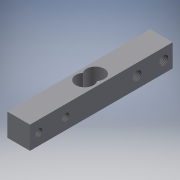
# Autodesk Inventor part: Celda
Saved by Autodesk Inventor 2019 (Build 230136000, 136)
## iProperties
Created: 2020-01-19
Part Number: Celda
Material: Generic
Document SubType Name: Modeling
Designer: peter
Density: 2.69895 g/cm^3
Appearance: Default
Mass: 28 g
Surface Area: 52.6894 cm^2
Volume: 10.3744 cm^3
Author: peter
Autodesk Inventor part; units mm, degrees
ref_plane "YZ Plane" through (0, 0, 0) normal (1, 0, 0) x (0, 1, 0)
ref_plane "XZ Plane" through (0, 0, 0) normal (0, 1, 0) x (-1, 0, 0)
ref_plane "XY Plane" through (0, 0, 0) normal (0, 0, 1) x (1, 0, 0)
sketch "Sketch1" plane through (0, 0, 0) normal (0, 1, 0) x (-1, 0, 0)
  line L0 (9.5195, 30.881) -> (-3.1805, 30.881)
  line L1 (-3.1805, 30.881) -> (-3.1805, -49.119)
  line L2 (-3.1805, -49.119) -> (9.5195, -49.119)
  line L3 (9.5195, -49.119) -> (9.5195, 30.881)
  arc A0 (-0.8493, -9.119) -> (7.1507, -9.119) centre (3.1507, -12.119) ccw
  arc A1 (7.1507, -9.119) -> (-0.8493, -9.119) centre (3.1507, -6.119) ccw
  point P0 (0, 0)
  dimension "d0" = 80
  dimension "d1" = 12.7
  constraints: 8 end point, 4 point on circle, 2 centre point, 2 parallel, 1 horizontal, 1 perpendicular
  measures "d0" distance of L2.end L0.start
  measures "d1" distance of L0.end L0.start
extrude "Extrusion1" add sketch "Sketch1" along normal blind 12.7
sketch "Sketch2" plane through (3.1805, 0, 30.881) normal (1, 0, 0) x (0, 0, -1)
  circle A0 centre (20, 6.35) radius 2
  line L0 (40, 0) -> (40, 12.7) projected
  line L1 (0, 0) -> (80, 0) projected
  circle A1 centre (5, 6.35) radius 2
  circle A2 centre (60, 6.35) radius 2.5
  circle A3 centre (75, 6.35) radius 2.5
  line L2 (80, 0) -> (80, 12.7) projected
  line L3 (0, 0) -> (0, 12.7) projected
  point P0 (30.881, 0)
  dimension "d7" = 4
  dimension "d9" = 20
  dimension "d11" = 6.35
  dimension "d12" = 4
  dimension "d13" = 15
  dimension "d14" = 6.35
  dimension "d16" = 5
  dimension "d17" = 20
  dimension "d18" = 6.35
  dimension "d19" = 5
  dimension "d20" = 15
  constraints: 4 centre point
  measures "d7" diameter of A0
  measures "d9" distance from line of L0 A0.centre
  measures "d11" distance from line of L1 A0.centre
  measures "d12" diameter of A1
  measures "d13" distance of A1.centre A0.centre
  measures "d14" distance from line of L1 A1.centre
  measures "d16" diameter of A2
  measures "d17" distance from line of L0 A2.centre
  measures "d18" distance from line of L1 A2.centre
  measures "d19" diameter of A3
  measures "d20" distance of A3.centre A2.centre
extrude "Extrusion2" cut sketch "Sketch2" against normal blind 12.7
thread "Thread1" size "M4x0.7" class "6H" standard "ISO Metric profile" full length
thread "Thread2" size "M4x0.7" class "6H" standard "ANSI Metric M Profile" full length
thread "Thread3" size "M5x0.8" class "6H" standard "ANSI Metric M Profile" full length
thread "Thread4" size "M5x0.8" class "6H" standard "ANSI Metric M Profile" full length
body "Solid1"
